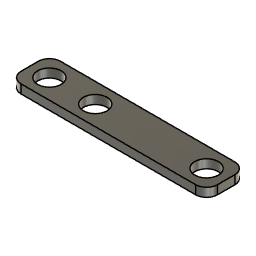
L1.3 (Autodesk Fusion 360 design; units mm, degrees)
Autodesk Fusion 360 part; units mm, degrees
sketch "Sketch1" plane through (0, 0, 0) normal (0, 0, 1) x (1, 0, 0)
  line L0 (22.5, 4.5) -> (-22.5, 4.5)
  line L1 (-22.5, 4.5) -> (-22.5, -4.5)
  line L2 (-22.5, -4.5) -> (22.5, -4.5)
  line L3 (22.5, -4.5) -> (22.5, 4.5)
  line L4 (22.5, 4.5) -> (-22.5, -4.5) construction
  line L5 (-22.5, 4.5) -> (22.5, -4.5) construction
  dimension "d1" = 45
  dimension "d2" = 9
  constraint horizontal L0
  constraint perpendicular L0 L1
  constraint parallel L0 L2
  constraint parallel L1 L3
  constraint coincident L4 origin
  constraint coincident L5 origin
  measures "d1" distance of L1.end L2.end
  measures "d2" distance of L0.end L1.end
extrude "Extrude1" add sketch "Sketch1" along normal blind 2
fillet "Fillet1" radius 2.5 4 edges at (-22.5, 4.5, 1) (-22.5, -4.5, 1) (22.5, -4.5, 1) (22.5, 4.5, 1)
sketch "Sketch2" plane through (0, 0, 2) normal (0, 0, 1) x (-1, 0, 0)
  arc A0 (-22.5, -2) -> (-20, -4.5) centre (-20, -2) ccw
  line L0 (-20, -4.5) -> (20, -4.5)
  arc A1 (22.5, 2) -> (20, 4.5) centre (20, 2) ccw
  line L1 (20, 4.5) -> (-20, 4.5)
  arc A2 (20, -4.5) -> (22.5, -2) centre (20, -2) ccw
  line L2 (22.5, -2) -> (22.5, 2)
  arc A3 (-20, 4.5) -> (-22.5, 2) centre (-20, 2) ccw
  line L3 (-22.5, 2) -> (-22.5, -2)
  line L4 (22.5, 0) -> (-22.5, 0) construction
  line L5 (22.5, 0) -> (18, 0)
  line L6 (-22.5, 0) -> (-18, 0)
  circle A4 centre (18, 0) radius 2.7
  circle A5 centre (-18, 0) radius 2.7
  dimension "d15" = 4.5
  dimension "d16" = 4.5
  dimension "d17" = 5.4
  dimension "d18" = 5.4
  constraint midpoint L2 L4.start
  constraint midpoint L3 L4.end
  constraint perpendicular L2 L5
  constraint perpendicular L3 L6
  constraint coincident L5.end A4.centre
  constraint coincident L6.end A5.centre
  measures "d15" distance of L4.start L5.end
  measures "d16" distance of L4.end L6.end
  measures "d17" diameter of A4
  measures "d18" diameter of A5
extrude "Extrude2" cut sketch "Sketch2" against normal blind 3 contours A4 | A5
sketch "Sketch3" plane through (0, 0, 2) normal (0, 0, 1) x (-1, 0, 0)
  arc A0 (-22.5, -2) -> (-20, -4.5) centre (-20, -2) ccw
  line L0 (-20, -4.5) -> (20, -4.5)
  arc A1 (22.5, 2) -> (20, 4.5) centre (20, 2) ccw
  line L1 (20, 4.5) -> (-20, 4.5)
  arc A2 (20, -4.5) -> (22.5, -2) centre (20, -2) ccw
  line L2 (22.5, -2) -> (22.5, 2)
  arc A3 (-20, 4.5) -> (-22.5, 2) centre (-20, 2) ccw
  line L3 (-22.5, 2) -> (-22.5, -2)
  circle A4 centre (18, 0) radius 2.7
  circle A5 centre (-18, 0) radius 2.7
  line L4 (22.5, 0) -> (-22.5, 0) construction
  line L5 (22.5, 0) -> (7.5, 0)
  circle A6 centre (7.5, 0) radius 2.7
  dimension "d19" = 15
  dimension "d20" = 5.4
  constraint midpoint L2 L4.start
  constraint midpoint L3 L4.end
  constraint perpendicular L2 L5
  constraint coincident L5.end A6.centre
  measures "d19" distance of L4.start L5.end
  measures "d20" diameter of A6
extrude "Extrude3" cut sketch "Sketch3" against normal blind 2 contours A6
